Autodesk Fusion 360 part; units mm, degrees
(part 2 of 3)
  arc A296 (115.4627, 116.2428) -> (115.5827, 116.3629) centre (115.4627, 116.3629) ccw
  arc A297 (96.7858, 84.677) -> (96.862, 84.7532) centre (96.7858, 84.7532) ccw
  arc A298 (57.1697, 56.4515) -> (57.2897, 56.5715) centre (57.1697, 56.5715) ccw
  arc A299 (113.2577, 58.5983) -> (113.3777, 58.7183) centre (113.2577, 58.7183) ccw
  line L491 (67.31, 68.0838) -> (67.31, 67.2202)
  line L492 (57.2897, 59.4163) -> (57.2897, 60.7765)
  arc A300 (50.1015, 56.3683) -> (50.2215, 56.2483) centre (50.2215, 56.3683) ccw
  arc A301 (115.5827, 117.9262) -> (115.4627, 118.0462) centre (115.4627, 117.9262) ccw
  line L493 (115.5391, 123.5075) -> (113.9758, 123.5075)
  line L494 (113.9758, 119.0625) -> (115.5391, 119.0625)
  arc A302 (105.1869, 119.9007) -> (105.0668, 119.7807) centre (105.1869, 119.7807) ccw
  line L495 (50.1015, 57.9317) -> (50.1015, 56.3683)
  arc A303 (106.667, 119.7807) -> (106.547, 119.9007) centre (106.547, 119.7807) ccw
  line L496 (55.4863, 57.9317) -> (55.4863, 56.5715)
  line L497 (96.862, 84.7532) -> (96.862, 85.6168)
  arc A304 (105.0668, 118.2173) -> (105.1869, 118.0973) centre (105.1869, 118.2173) ccw
  arc A305 (115.5391, 119.0625) -> (115.6592, 119.1825) centre (115.5391, 119.1825) ccw
  arc A306 (68.326, 66.3838) -> (68.2498, 66.46) centre (68.2498, 66.3838) ccw
  arc A307 (113.9758, 120.6627) -> (113.8558, 120.5427) centre (113.9758, 120.5427) ccw
  line L498 (113.8558, 123.3875) -> (113.8558, 122.0273)
  line L499 (111.7775, 60.2817) -> (111.7775, 58.7183)
  line L500 (113.2577, 60.4017) -> (111.8975, 60.4017)
  line L501 (114.6223, 60.2817) -> (114.6223, 58.7183)
  arc A308 (95.846, 84.7532) -> (95.9222, 84.677) centre (95.9222, 84.7532) ccw
  line L502 (57.1697, 60.8965) -> (55.6063, 60.8965)
  line L503 (115.5827, 116.3629) -> (115.5827, 117.9262)
  line L504 (111.8975, 58.5983) -> (113.2577, 58.5983)
  line L505 (113.9825, 117.9262) -> (113.9825, 116.3629)
  line L506 (96.7858, 85.693) -> (95.9222, 85.693)
  line L507 (108.1532, 114.5165) -> (109.0168, 114.5165)
  arc A309 (57.2897, 57.9317) -> (57.1697, 58.0517) centre (57.1697, 57.9317) ccw
  line L508 (109.0168, 115.5325) -> (108.1532, 115.5325)
  arc A310 (111.8975, 60.4017) -> (111.7775, 60.2817) centre (111.8975, 60.2817) ccw
  arc A311 (95.9222, 85.693) -> (95.846, 85.6168) centre (95.9222, 85.6168) ccw
  line L509 (95.0858, 85.693) -> (94.2222, 85.693)
  arc A312 (113.9825, 116.3629) -> (114.1025, 116.2428) centre (114.1025, 116.3629) ccw
  line L510 (51.5817, 58.0517) -> (50.2215, 58.0517)
  arc A313 (115.5391, 121.9073) -> (115.6592, 122.0273) centre (115.5391, 122.0273) ccw
  line L511 (109.093, 114.5927) -> (109.093, 115.4563)
  arc A314 (108.1532, 115.5325) -> (108.077, 115.4563) centre (108.1532, 115.4563) ccw
  arc A315 (57.1697, 59.2963) -> (57.2897, 59.4163) centre (57.1697, 59.4163) ccw
  arc A316 (108.077, 114.5927) -> (108.1532, 114.5165) centre (108.1532, 114.5927) ccw
  arc A317 (109.0168, 114.5165) -> (109.093, 114.5927) centre (109.0168, 114.5927) ccw
  line L512 (95.846, 85.6168) -> (95.846, 84.7532)
  line L513 (118.4275, 116.3629) -> (118.4275, 117.9262)
  line L514 (57.2897, 56.5715) -> (57.2897, 57.9317)
  arc A318 (109.093, 115.4563) -> (109.0168, 115.5325) centre (109.0168, 115.4563) ccw
  arc A319 (96.862, 85.6168) -> (96.7858, 85.693) centre (96.7858, 85.6168) ccw
  arc A320 (95.0858, 84.677) -> (95.162, 84.7532) centre (95.0858, 84.7532) ccw
  arc A321 (55.6063, 60.8965) -> (55.4863, 60.7765) centre (55.6063, 60.7765) ccw
  arc A322 (57.2897, 60.7765) -> (57.1697, 60.8965) centre (57.1697, 60.7765) ccw
  arc A323 (116.9473, 118.0462) -> (116.8273, 117.9262) centre (116.9473, 117.9262) ccw
  line L515 (108.1532, 116.2165) -> (109.0168, 116.2165)
  arc A324 (68.2498, 67.144) -> (68.326, 67.2202) centre (68.2498, 67.2202) ccw
  arc A325 (94.146, 84.7532) -> (94.2222, 84.677) centre (94.2222, 84.7532) ccw
  line L516 (68.2498, 68.16) -> (67.3862, 68.16)
  arc A326 (67.31, 65.5202) -> (67.3862, 65.444) centre (67.3862, 65.5202) ccw
  arc A327 (55.6063, 58.0517) -> (55.4863, 57.9317) centre (55.6063, 57.9317) ccw
  arc A328 (111.6705, 112.3188) -> (111.5943, 112.395) centre (111.5943, 112.3188) ccw
  arc A329 (109.0168, 116.2165) -> (109.093, 116.2927) centre (109.0168, 116.2927) ccw
  line L517 (108.9545, 112.3188) -> (108.9545, 111.4552)
  arc A330 (55.4863, 59.4163) -> (55.6063, 59.2963) centre (55.6063, 59.4163) ccw
  line L518 (107.149, 112.3188) -> (107.149, 111.4552)
  line L519 (116.0662, 111.379) -> (116.9298, 111.379)
  line L520 (68.2498, 66.46) -> (67.3862, 66.46)
  arc A331 (117.006, 112.3188) -> (116.9298, 112.395) centre (116.9298, 112.3188) ccw
  line L521 (55.6063, 56.4515) -> (57.1697, 56.4515)
  line L522 (57.1697, 58.0517) -> (55.6063, 58.0517)
  arc A332 (108.1532, 117.2325) -> (108.077, 117.1563) centre (108.1532, 117.1563) ccw
  line L523 (118.706, 111.4552) -> (118.706, 112.3188)
  arc A333 (106.465, 112.3188) -> (106.3888, 112.395) centre (106.3888, 112.3188) ccw
  arc A334 (68.326, 68.0838) -> (68.2498, 68.16) centre (68.2498, 68.0838) ccw
  line L524 (50.2215, 56.2483) -> (51.5817, 56.2483)
  line L525 (95.9222, 84.677) -> (96.7858, 84.677)
  line L526 (55.4863, 60.7765) -> (55.4863, 59.4163)
  arc A335 (109.093, 117.1563) -> (109.0168, 117.2325) centre (109.0168, 117.1563) ccw
  arc A336 (51.7017, 57.9317) -> (51.5817, 58.0517) centre (51.5817, 57.9317) ccw
  line L527 (114.2361, 111.379) -> (115.0997, 111.379)
  line L528 (115.1759, 111.4552) -> (115.1759, 112.3188)
  arc A337 (67.3862, 68.16) -> (67.31, 68.0838) centre (67.3862, 68.0838) ccw
  arc A338 (51.5817, 56.2483) -> (51.7017, 56.3683) centre (51.5817, 56.3683) ccw
  line L529 (114.1599, 112.3188) -> (114.1599, 111.4552)
  arc A339 (67.31, 67.2202) -> (67.3862, 67.144) centre (67.3862, 67.2202) ccw
  arc A340 (115.0997, 111.379) -> (115.1759, 111.4552) centre (115.0997, 111.4552) ccw
  line L530 (108.077, 117.1563) -> (108.077, 116.2927)
  line L531 (67.31, 66.3838) -> (67.31, 65.5202)
  line L532 (94.146, 85.6168) -> (94.146, 84.7532)
  arc A341 (108.165, 112.3188) -> (108.0888, 112.395) centre (108.0888, 112.3188) ccw
  line L533 (109.9705, 111.4552) -> (109.9705, 112.3188)
  arc A342 (55.4863, 56.5715) -> (55.6063, 56.4515) centre (55.6063, 56.5715) ccw
  line L534 (68.326, 67.2202) -> (68.326, 68.0838)
  arc A343 (67.3862, 66.46) -> (67.31, 66.3838) centre (67.3862, 66.3838) ccw
  arc A344 (116.0662, 112.395) -> (115.99, 112.3188) centre (116.0662, 112.3188) ccw
  arc A345 (115.1759, 112.3188) -> (115.0997, 112.395) centre (115.0997, 112.3188) ccw
  arc A346 (114.1599, 111.4552) -> (114.2361, 111.379) centre (114.2361, 111.4552) ccw
  line L535 (110.7307, 111.379) -> (111.5943, 111.379)
  line L536 (55.6063, 59.2963) -> (57.1697, 59.2963)
  line L537 (107.2252, 111.379) -> (108.0888, 111.379)
  line L538 (117.7662, 111.379) -> (118.6298, 111.379)
  line L539 (67.3862, 65.444) -> (68.2498, 65.444)
  arc A347 (109.0307, 112.395) -> (108.9545, 112.3188) centre (109.0307, 112.3188) ccw
  line L540 (108.165, 111.4552) -> (108.165, 112.3188)
  arc A348 (94.2222, 85.693) -> (94.146, 85.6168) centre (94.2222, 85.6168) ccw
  line L541 (115.0997, 112.395) -> (114.2361, 112.395)
  arc A349 (68.2498, 65.444) -> (68.326, 65.5202) centre (68.2498, 65.5202) ccw
  line L542 (108.0888, 112.395) -> (107.2252, 112.395)
  line L543 (118.6298, 112.395) -> (117.7662, 112.395)
  arc A350 (114.2361, 112.395) -> (114.1599, 112.3188) centre (114.2361, 112.3188) ccw
  arc A351 (50.2215, 58.0517) -> (50.1015, 57.9317) centre (50.2215, 57.9317) ccw
  line L544 (115.99, 112.3188) -> (115.99, 111.4552)
  line L545 (117.006, 111.4552) -> (117.006, 112.3188)
  line L546 (116.9298, 112.395) -> (116.0662, 112.395)
  line L547 (109.0307, 111.379) -> (109.8943, 111.379)
  line L548 (95.162, 84.7532) -> (95.162, 85.6168)
  line L549 (105.5252, 111.379) -> (106.3888, 111.379)
  line L550 (68.326, 65.5202) -> (68.326, 66.3838)
  arc A352 (93.2688, 79.001) -> (93.345, 79.0772) centre (93.2688, 79.0772) ccw
  line L551 (105.449, 112.3188) -> (105.449, 111.4552)
  arc A353 (93.2688, 80.701) -> (93.345, 80.7772) centre (93.2688, 80.7772) ccw
  arc A354 (117.69, 111.4552) -> (117.7662, 111.379) centre (117.7662, 111.4552) ccw
  arc A355 (115.99, 111.4552) -> (116.0662, 111.379) centre (116.0662, 111.4552) ccw
  arc A356 (59.182, 50.4562) -> (59.2582, 50.38) centre (59.2582, 50.4562) ccw
  line L552 (109.093, 116.2927) -> (109.093, 117.1563)
  line L553 (113.4759, 111.4552) -> (113.4759, 112.3188)
  arc A357 (116.9298, 111.379) -> (117.006, 111.4552) centre (116.9298, 111.4552) ccw
  arc A358 (45.9622, 85.725) -> (45.886, 85.6488) centre (45.9622, 85.6488) ccw
  arc A359 (112.5361, 112.395) -> (112.4599, 112.3188) centre (112.5361, 112.3188) ccw
  arc A360 (113.4759, 112.3188) -> (113.3997, 112.395) centre (113.3997, 112.3188) ccw
  line L554 (106.465, 111.4552) -> (106.465, 112.3188)
  arc A361 (111.5943, 111.379) -> (111.6705, 111.4552) centre (111.5943, 111.4552) ccw
  line L555 (92.4052, 79.001) -> (93.2688, 79.001)
  arc A362 (93.345, 79.9408) -> (93.2688, 80.017) centre (93.2688, 79.9408) ccw
  arc A363 (60.1218, 50.38) -> (60.198, 50.4562) centre (60.1218, 50.4562) ccw
  arc A364 (105.449, 111.4552) -> (105.5252, 111.379) centre (105.5252, 111.4552) ccw
  line L556 (60.198, 48.7562) -> (60.198, 49.6198)
  arc A365 (118.706, 112.3188) -> (118.6298, 112.395) centre (118.6298, 112.3188) ccw
  line L557 (112.5361, 111.379) -> (113.3997, 111.379)
  line L558 (110.6545, 112.3188) -> (110.6545, 111.4552)
  arc A366 (109.9705, 112.3188) -> (109.8943, 112.395) centre (109.8943, 112.3188) ccw
  arc A367 (105.5252, 112.395) -> (105.449, 112.3188) centre (105.5252, 112.3188) ccw
  line L559 (47.586, 85.6488) -> (47.586, 84.7852)
  arc A368 (107.149, 111.4552) -> (107.2252, 111.379) centre (107.2252, 111.4552) ccw
  line L560 (92.329, 79.9408) -> (92.329, 79.0772)
  arc A369 (110.7307, 112.395) -> (110.6545, 112.3188) centre (110.7307, 112.3188) ccw
  arc A370 (48.5258, 84.709) -> (48.602, 84.7852) centre (48.5258, 84.7852) ccw
  line L561 (117.69, 112.3188) -> (117.69, 111.4552)
  arc A371 (108.077, 116.2927) -> (108.1532, 116.2165) centre (108.1532, 116.2927) ccw
  arc A372 (92.4052, 84.081) -> (92.329, 84.0048) centre (92.4052, 84.0048) ccw
  arc A373 (47.6622, 85.725) -> (47.586, 85.6488) centre (47.6622, 85.6488) ccw
  line L562 (92.329, 81.6408) -> (92.329, 80.7772)
  line L563 (60.1218, 51.396) -> (59.2582, 51.396)
  line L564 (93.345, 83.1412) -> (93.345, 84.0048)
  line L565 (59.2582, 50.38) -> (60.1218, 50.38)
  arc A374 (118.6298, 111.379) -> (118.706, 111.4552) centre (118.6298, 111.4552) ccw
  line L566 (111.5943, 112.395) -> (110.7307, 112.395)
  line L567 (109.8943, 112.395) -> (109.0307, 112.395)
  line L568 (92.329, 85.7048) -> (92.329, 84.8412)
  line L569 (93.345, 80.7772) -> (93.345, 81.6408)
  arc A375 (60.198, 51.3198) -> (60.1218, 51.396) centre (60.1218, 51.3198) ccw
  arc A376 (108.9545, 111.4552) -> (109.0307, 111.379) centre (109.0307, 111.4552) ccw
  arc A377 (110.6545, 111.4552) -> (110.7307, 111.379) centre (110.7307, 111.4552) ccw
  line L570 (47.6622, 84.709) -> (48.5258, 84.709)
  line L571 (109.0168, 117.2325) -> (108.1532, 117.2325)
  arc A378 (92.329, 84.8412) -> (92.4052, 84.765) centre (92.4052, 84.8412) ccw
  arc A379 (59.2582, 51.396) -> (59.182, 51.3198) centre (59.2582, 51.3198) ccw
  line L572 (111.6705, 111.4552) -> (111.6705, 112.3188)
  arc A380 (107.2252, 112.395) -> (107.149, 112.3188) centre (107.2252, 112.3188) ccw
  arc A381 (108.0888, 111.379) -> (108.165, 111.4552) centre (108.0888, 111.4552) ccw
  arc A382 (117.7662, 112.395) -> (117.69, 112.3188) centre (117.7662, 112.3188) ccw
  arc A383 (92.329, 80.7772) -> (92.4052, 80.701) centre (92.4052, 80.7772) ccw
  line L573 (46.902, 84.7852) -> (46.902, 85.6488)
  line L574 (59.182, 51.3198) -> (59.182, 50.4562)
  arc A384 (106.3888, 111.379) -> (106.465, 111.4552) centre (106.3888, 111.4552) ccw
  line L575 (60.198, 50.4562) -> (60.198, 51.3198)
  arc A385 (92.4052, 81.717) -> (92.329, 81.6408) centre (92.4052, 81.6408) ccw
  line L576 (106.3888, 112.395) -> (105.5252, 112.395)
  line L577 (93.2688, 81.717) -> (92.4052, 81.717)
  arc A386 (109.8943, 111.379) -> (109.9705, 111.4552) centre (109.8943, 111.4552) ccw
  line L578 (58.711, 77.262) -> (58.711, 76.662)
  line L579 (53.811, 77.262) -> (52.211, 77.262)
  line L580 (52.211, 77.262) -> (52.211, 76.662)
  arc A387 (105.456, 63.44) -> (104.856, 63.44) centre (105.156, 63.44) ccw
  line L581 (105.456, 57.24) -> (104.856, 57.24)
  line L582 (107.996, 57.24) -> (107.396, 57.24)
  line L583 (104.856, 57.24) -> (104.856, 55.64)
  line L584 (107.996, 55.64) -> (107.996, 57.24)
  line L585 (107.396, 57.24) -> (107.396, 55.64)
  line L586 (107.996, 63.74) -> (107.396, 63.74)
  line L587 (53.811, 76.662) -> (53.811, 77.262)
  line L588 (53.511, 74.722) -> (52.511, 74.722)
  line L589 (97.5478, 65.659) -> (96.6842, 65.659)
  line L590 (96.608, 65.5828) -> (96.608, 64.7192)
  line L591 (107.396, 55.64) -> (107.996, 55.64)
  arc A388 (96.608, 64.7192) -> (96.6842, 64.643) centre (96.6842, 64.7192) ccw
  line L592 (60.311, 77.262) -> (58.711, 77.262)
  line L593 (107.996, 62.14) -> (107.996, 63.74)
  line L594 (60.311, 74.122) -> (60.311, 74.722)
  line L595 (104.856, 62.44) -> (104.856, 63.44)
  line L596 (105.456, 62.44) -> (105.456, 63.44)
  line L597 (104.856, 55.64) -> (105.456, 55.64)
  line L598 (58.711, 74.122) -> (60.311, 74.122)
  line L599 (60.311, 74.722) -> (58.711, 74.722)
  line L600 (52.211, 76.662) -> (53.811, 76.662)
  arc A389 (52.511, 74.722) -> (52.511, 74.122) centre (52.511, 74.422) ccw
  line L601 (107.396, 62.14) -> (107.996, 62.14)
  line L602 (107.396, 63.74) -> (107.396, 62.14)
  line L603 (105.456, 55.64) -> (105.456, 57.24)
  line L604 (58.711, 74.722) -> (58.711, 74.122)
  line L605 (106.0078, 65.532) -> (105.1442, 65.532)
  line L606 (97.624, 64.7192) -> (97.624, 65.5828)
  arc A390 (94.322, 65.5828) -> (94.2458, 65.659) centre (94.2458, 65.5828) ccw
  arc A391 (97.5478, 64.643) -> (97.624, 64.7192) centre (97.5478, 64.7192) ccw
  line L607 (91.6822, 64.643) -> (92.5458, 64.643)
  arc A392 (94.9842, 65.659) -> (94.908, 65.5828) centre (94.9842, 65.5828) ccw
  line L608 (105.1442, 64.516) -> (106.0078, 64.516)
  arc A393 (106.768, 64.5922) -> (106.8442, 64.516) centre (106.8442, 64.5922) ccw
  line L609 (104.355, 64.5922) -> (104.355, 65.4558)
  line L610 (93.306, 65.5828) -> (93.306, 64.7192)
  line L611 (103.4152, 64.516) -> (104.2788, 64.516)
  arc A394 (106.084, 65.4558) -> (106.0078, 65.532) centre (106.0078, 65.4558) ccw
  line L612 (92.5458, 65.659) -> (91.6822, 65.659)
  arc A395 (91.606, 64.7192) -> (91.6822, 64.643) centre (91.6822, 64.7192) ccw
  arc A396 (92.622, 65.5828) -> (92.5458, 65.659) centre (92.5458, 65.5828) ccw
  arc A397 (95.8478, 64.643) -> (95.924, 64.7192) centre (95.8478, 64.7192) ccw
  line L613 (106.8442, 64.516) -> (107.7078, 64.516)
  line L614 (107.784, 64.5922) -> (107.784, 65.4558)
  arc A398 (107.7078, 64.516) -> (107.784, 64.5922) centre (107.7078, 64.5922) ccw
  arc A399 (97.624, 65.5828) -> (97.5478, 65.659) centre (97.5478, 65.5828) ccw
  arc A400 (93.306, 64.7192) -> (93.3822, 64.643) centre (93.3822, 64.7192) ccw
  arc A401 (94.908, 64.7192) -> (94.9842, 64.643) centre (94.9842, 64.7192) ccw
  line L615 (94.908, 65.5828) -> (94.908, 64.7192)
  arc A402 (106.8442, 65.532) -> (106.768, 65.4558) centre (106.8442, 65.4558) ccw
  arc A403 (95.924, 65.5828) -> (95.8478, 65.659) centre (95.8478, 65.5828) ccw
  line L616 (103.339, 65.4558) -> (103.339, 64.5922)
  arc A404 (106.0078, 64.516) -> (106.084, 64.5922) centre (106.0078, 64.5922) ccw
  line L617 (94.2458, 65.659) -> (93.3822, 65.659)
  line L618 (95.8478, 65.659) -> (94.9842, 65.659)
  line L619 (93.3822, 64.643) -> (94.2458, 64.643)
  line L620 (104.2788, 65.532) -> (103.4152, 65.532)
  arc A405 (96.6842, 65.659) -> (96.608, 65.5828) centre (96.6842, 65.5828) ccw
  line L621 (101.639, 65.4558) -> (101.639, 64.5922)
  arc A406 (93.3822, 65.659) -> (93.306, 65.5828) centre (93.3822, 65.5828) ccw
  arc A407 (103.339, 64.5922) -> (103.4152, 64.516) centre (103.4152, 64.5922) ccw
  arc A408 (102.655, 65.4558) -> (102.5788, 65.532) centre (102.5788, 65.4558) ccw
  arc A409 (94.2458, 64.643) -> (94.322, 64.7192) centre (94.2458, 64.7192) ccw
  line L622 (94.322, 64.7192) -> (94.322, 65.5828)
  line L623 (92.622, 64.7192) -> (92.622, 65.5828)
  line L624 (102.5788, 65.532) -> (101.7152, 65.532)
  arc A410 (105.1442, 65.532) -> (105.068, 65.4558) centre (105.1442, 65.4558) ccw
  arc A411 (101.639, 64.5922) -> (101.7152, 64.516) centre (101.7152, 64.5922) ccw
  line L625 (94.9842, 64.643) -> (95.8478, 64.643)
  arc A412 (107.784, 65.4558) -> (107.7078, 65.532) centre (107.7078, 65.4558) ccw
  line L626 (101.7152, 64.516) -> (102.5788, 64.516)
  arc A413 (91.6822, 65.659) -> (91.606, 65.5828) centre (91.6822, 65.5828) ccw
  arc A414 (104.2788, 64.516) -> (104.355, 64.5922) centre (104.2788, 64.5922) ccw
  line L627 (95.141, 48.71) -> (94.741, 49.11)
  line L628 (107.7078, 65.532) -> (106.8442, 65.532)
  arc A415 (104.355, 65.4558) -> (104.2788, 65.532) centre (104.2788, 65.4558) ccw
  line L629 (91.606, 65.5828) -> (91.606, 64.7192)
  line L630 (102.655, 64.5922) -> (102.655, 65.4558)
  arc A416 (105.068, 64.5922) -> (105.1442, 64.516) centre (105.1442, 64.5922) ccw
  arc A417 (103.4152, 65.532) -> (103.339, 65.4558) centre (103.4152, 65.4558) ccw
  line L631 (95.924, 64.7192) -> (95.924, 65.5828)
  arc A418 (101.7152, 65.532) -> (101.639, 65.4558) centre (101.7152, 65.4558) ccw
  line L632 (105.068, 65.4558) -> (105.068, 64.5922)
  line L633 (106.768, 65.4558) -> (106.768, 64.5922)
  arc A419 (92.5458, 64.643) -> (92.622, 64.7192) centre (92.5458, 64.7192) ccw
  line L634 (106.084, 64.5922) -> (106.084, 65.4558)
  line L635 (96.6842, 64.643) -> (97.5478, 64.643)
  arc A420 (51.8042, 50.419) -> (51.728, 50.3428) centre (51.8042, 50.3428) ccw
  line L636 (55.303, 51.1585) -> (55.5155, 50.946)
  line L637 (55.9905, 51.796) -> (55.5155, 51.796)
  line L638 (55.303, 51.5835) -> (55.303, 51.1585)
  line L639 (55.5155, 50.946) -> (55.9905, 50.946)
  line L640 (93.941, 49.11) -> (93.541, 48.71)
  line L641 (93.941, 47.41) -> (94.741, 47.41)
  line L642 (55.9905, 50.946) -> (56.203, 51.1585)
  line L643 (56.203, 51.1585) -> (56.203, 51.5835)
  line L644 (109.151, 47.41) -> (109.151, 49.11)
  line L645 (116.389, 67.157) -> (116.389, 70.257)
  line L646 (97.391, 49.11) -> (97.391, 47.41)
  line L647 (93.541, 47.81) -> (93.941, 47.41)
  line L648 (52.6678, 50.419) -> (51.8042, 50.419)
  line L649 (51.728, 50.3428) -> (51.728, 49.4792)
  line L650 (93.541, 48.71) -> (93.541, 47.81)
  arc A421 (53.428, 49.4792) -> (53.5042, 49.403) centre (53.5042, 49.4792) ccw
  arc A422 (51.728, 49.4792) -> (51.8042, 49.403) centre (51.8042, 49.4792) ccw
  line L651 (54.444, 49.4792) -> (54.444, 50.3428)
  line L652 (107.551, 47.41) -> (109.151, 47.41)
  line L653 (104.101, 47.41) -> (104.901, 47.41)
  line L654 (52.744, 49.4792) -> (52.744, 50.3428)
  line L655 (51.8042, 49.403) -> (52.6678, 49.403)
  arc A423 (52.6678, 49.403) -> (52.744, 49.4792) centre (52.6678, 49.4792) ccw
  arc A424 (54.444, 50.3428) -> (54.3678, 50.419) centre (54.3678, 50.3428) ccw
  line L656 (103.701, 48.71) -> (103.701, 47.81)
  line L657 (95.141, 47.81) -> (95.141, 48.71)
  arc A425 (53.5042, 50.419) -> (53.428, 50.3428) centre (53.5042, 50.3428) ccw
  line L658 (55.303, 49.296) -> (56.203, 49.296)
  line L659 (55.303, 50.146) -> (55.303, 49.296)
  line L660 (55.5155, 51.796) -> (55.303, 51.5835)
  line L661 (54.3678, 50.419) -> (53.5042, 50.419)
  line L662 (113.989, 70.257) -> (113.989, 67.157)
  arc A426 (54.3678, 49.403) -> (54.444, 49.4792) centre (54.3678, 49.4792) ccw
  line L663 (104.901, 47.41) -> (105.301, 47.81)
  arc A427 (102.5788, 64.516) -> (102.655, 64.5922) centre (102.5788, 64.5922) ccw
  line L664 (94.741, 49.11) -> (93.941, 49.11)
  line L665 (117.014, 69.642) -> (117.014, 69.042)
  line L666 (53.428, 50.3428) -> (53.428, 49.4792)
  line L667 (118.764, 70.312) -> (118.764, 70.912)
  line L668 (118.764, 69.642) -> (117.014, 69.642)
  line L669 (117.014, 69.042) -> (118.764, 69.042)
  line L670 (113.989, 67.157) -> (116.389, 67.157)
  line L671 (118.764, 70.912) -> (117.014, 70.912)
  line L672 (53.5042, 49.403) -> (54.3678, 49.403)
  line L673 (103.701, 47.81) -> (104.101, 47.41)
  line L674 (98.991, 49.11) -> (97.391, 49.11)
  line L675 (56.203, 51.5835) -> (55.9905, 51.796)
  line L676 (56.203, 50.146) -> (55.303, 50.146)
  line L677 (98.991, 47.41) -> (98.991, 49.11)
  line L678 (97.391, 47.41) -> (98.991, 47.41)
  line L679 (117.014, 70.912) -> (117.014, 70.312)
  line L680 (105.301, 48.71) -> (104.901, 49.11)
  line L681 (107.551, 49.11) -> (107.551, 47.41)
  line L682 (118.764, 69.042) -> (118.764, 69.642)
  line L683 (116.389, 70.257) -> (113.989, 70.257)
  line L684 (109.151, 49.11) -> (107.551, 49.11)
  line L685 (104.901, 49.11) -> (104.101, 49.11)
  line L686 (56.203, 49.296) -> (56.203, 50.146)
  line L687 (117.014, 70.312) -> (118.764, 70.312)
  line L688 (104.101, 49.11) -> (103.701, 48.71)
  arc A428 (52.744, 50.3428) -> (52.6678, 50.419) centre (52.6678, 50.3428) ccw
  line L689 (105.301, 47.81) -> (105.301, 48.71)
  line L690 (94.741, 47.41) -> (95.141, 47.81)
  arc A429 (93.0402, 70.954) -> (92.964, 70.8778) centre (93.0402, 70.8778) ccw
  line L691 (118.764, 67.102) -> (117.014, 67.102)
  line L692 (111.614, 68.372) -> (111.614, 67.772)
  line L693 (111.614, 70.912) -> (111.614, 70.312)
  line L694 (113.064, 66.502) -> (111.914, 66.502)
  line L695 (111.614, 70.312) -> (113.364, 70.312)
  line L696 (40.008, 63.7182) -> (40.008, 64.5818)
  line L697 (39.0682, 65.342) -> (39.9318, 65.342)
  arc A430 (39.9318, 65.342) -> (40.008, 65.4182) centre (39.9318, 65.4182) ccw
  line L698 (40.992, 66.2818) -> (40.992, 65.4182)
  line L699 (97.236, 63.74) -> (97.236, 62.14)
  line L700 (95.296, 57.24) -> (94.696, 57.24)
  line L701 (113.364, 68.372) -> (111.614, 68.372)
  line L702 (93.98, 70.0142) -> (93.98, 70.8778)
  line L703 (97.836, 62.14) -> (97.836, 63.74)
  line L704 (117.014, 67.772) -> (118.764, 67.772)
  arc A431 (42.008, 66.2818) -> (41.9318, 66.358) centre (41.9318, 66.2818) ccw
  line L705 (40.008, 65.4182) -> (40.008, 66.2818)
  arc A432 (40.992, 63.7182) -> (41.0682, 63.642) centre (41.0682, 63.7182) ccw
  line L706 (113.364, 70.912) -> (111.614, 70.912)
  line L707 (111.614, 69.642) -> (111.614, 69.042)
  line L708 (113.364, 69.042) -> (113.364, 69.642)
  arc A433 (53.511, 74.122) -> (53.511, 74.722) centre (53.511, 74.422) ccw
  line L709 (38.992, 66.2818) -> (38.992, 65.4182)
  line L710 (118.764, 66.502) -> (118.764, 67.102)
  line L711 (39.9318, 66.358) -> (39.0682, 66.358)
  line L712 (39.0682, 63.642) -> (39.9318, 63.642)
  line L713 (111.614, 69.042) -> (113.364, 69.042)
  line L714 (118.764, 67.772) -> (118.764, 68.372)
  line L715 (53.511, 74.122) -> (52.511, 74.122)
  line L716 (117.014, 66.502) -> (118.764, 66.502)
  arc A434 (39.0682, 66.358) -> (38.992, 66.2818) centre (39.0682, 66.2818) ccw
  line L717 (118.764, 68.372) -> (117.014, 68.372)
  line L718 (113.064, 67.102) -> (111.914, 67.102)
  line L719 (111.614, 67.772) -> (113.364, 67.772)
  line L720 (41.9318, 64.658) -> (41.0682, 64.658)
  line L721 (40.992, 64.5818) -> (40.992, 63.7182)
  line L722 (113.364, 69.642) -> (111.614, 69.642)
  line L723 (113.364, 70.312) -> (113.364, 70.912)
  line L724 (39.9318, 64.658) -> (39.0682, 64.658)
  line L725 (58.711, 76.662) -> (60.311, 76.662)
  line L726 (38.992, 64.5818) -> (38.992, 63.7182)
  arc A435 (40.008, 64.5818) -> (39.9318, 64.658) centre (39.9318, 64.5818) ccw
  line L727 (42.008, 63.7182) -> (42.008, 64.5818)
  line L728 (117.014, 68.372) -> (117.014, 67.772)
  arc A436 (40.008, 66.2818) -> (39.9318, 66.358) centre (39.9318, 66.2818) ccw
  line L729 (41.0682, 63.642) -> (41.9318, 63.642)
  line L730 (42.008, 65.4182) -> (42.008, 66.2818)
  line L731 (41.9318, 66.358) -> (41.0682, 66.358)
  arc A437 (111.914, 67.102) -> (111.914, 66.502) centre (111.914, 66.802) ccw
  arc A438 (41.0682, 66.358) -> (40.992, 66.2818) centre (41.0682, 66.2818) ccw
  arc A439 (113.064, 66.502) -> (113.064, 67.102) centre (113.064, 66.802) ccw
  line L732 (113.364, 67.772) -> (113.364, 68.372)
  arc A440 (38.992, 63.7182) -> (39.0682, 63.642) centre (39.0682, 63.7182) ccw
  arc A441 (38.992, 65.4182) -> (39.0682, 65.342) centre (39.0682, 65.4182) ccw
  line L733 (93.9038, 69.254) -> (93.0402, 69.254)
  arc A442 (93.98, 69.1778) -> (93.9038, 69.254) centre (93.9038, 69.1778) ccw
  arc A443 (95.296, 63.44) -> (94.696, 63.44) centre (94.996, 63.44) ccw
  arc A444 (39.0682, 64.658) -> (38.992, 64.5818) centre (39.0682, 64.5818) ccw
  arc A445 (41.0682, 64.658) -> (40.992, 64.5818) centre (41.0682, 64.5818) ccw
  line L734 (94.696, 55.64) -> (95.296, 55.64)
  arc A446 (39.9318, 63.642) -> (40.008, 63.7182) centre (39.9318, 63.7182) ccw
  arc A447 (41.9318, 65.342) -> (42.008, 65.4182) centre (41.9318, 65.4182) ccw
  line L735 (117.014, 67.102) -> (117.014, 66.502)
  arc A448 (61.722, 77.2532) -> (61.7982, 77.177) centre (61.7982, 77.2532) ccw
  line L736 (97.9873, 90.955) -> (97.8373, 91.105)
  line L737 (41.0682, 65.342) -> (41.9318, 65.342)
  line L738 (94.696, 62.44) -> (94.696, 63.44)
  line L739 (108.2873, 93.045) -> (108.2873, 93.645)
  line L740 (106.2373, 90.505) -> (108.2873, 90.505)
  line L741 (58.711, 80.98) -> (60.311, 80.98)
  arc A449 (61.722, 75.5532) -> (61.7982, 75.477) centre (61.7982, 75.5532) ccw
  line L742 (97.8373, 91.105) -> (96.0873, 91.105)
  line L743 (53.811, 84.12) -> (52.211, 84.12)
  line L744 (53.511, 80.98) -> (52.511, 80.98)
  line L745 (97.236, 57.24) -> (97.236, 55.64)
  arc A450 (92.964, 68.3142) -> (93.0402, 68.238) centre (93.0402, 68.3142) ccw
  line L746 (93.0402, 69.938) -> (93.9038, 69.938)
  arc A451 (104.856, 62.44) -> (105.456, 62.44) centre (105.156, 62.44) ccw
  line L747 (108.2873, 93.645) -> (106.2373, 93.645)
  line L748 (61.722, 76.4168) -> (61.722, 75.5532)
  arc A452 (61.7982, 76.493) -> (61.722, 76.4168) centre (61.7982, 76.4168) ccw
  arc A453 (52.511, 81.58) -> (52.511, 80.98) centre (52.511, 81.28) ccw
  line L749 (62.738, 77.2532) -> (62.738, 78.1168)
  arc A454 (62.6618, 75.477) -> (62.738, 75.5532) centre (62.6618, 75.5532) ccw
  line L750 (94.696, 57.24) -> (94.696, 55.64)
  line L751 (60.311, 81.58) -> (58.711, 81.58)
  arc A455 (62.738, 76.4168) -> (62.6618, 76.493) centre (62.6618, 76.4168) ccw
  line L752 (97.836, 57.24) -> (97.236, 57.24)
  line L753 (97.836, 55.64) -> (97.836, 57.24)
  line L754 (97.9873, 90.655) -> (97.9873, 90.955)
  line L755 (96.0873, 91.105) -> (95.9373, 90.955)
  line L756 (95.296, 55.64) -> (95.296, 57.24)
  line L757 (93.0402, 68.238) -> (93.9038, 68.238)
  line L758 (61.7982, 77.177) -> (62.6618, 77.177)
  arc A456 (93.9038, 69.938) -> (93.98, 70.0142) centre (93.9038, 70.0142) ccw
  arc A457 (53.511, 80.98) -> (53.511, 81.58) centre (53.511, 81.28) ccw
  line L759 (93.98, 68.3142) -> (93.98, 69.1778)
  line L760 (62.738, 75.5532) -> (62.738, 76.4168)
  line L761 (95.9373, 90.955) -> (95.9373, 90.655)
  arc A458 (93.9038, 68.238) -> (93.98, 68.3142) centre (93.9038, 68.3142) ccw
  arc A459 (93.98, 70.8778) -> (93.9038, 70.954) centre (93.9038, 70.8778) ccw
  line L762 (93.9038, 70.954) -> (93.0402, 70.954)
  line L763 (61.7982, 75.477) -> (62.6618, 75.477)
  arc A460 (41.9318, 63.642) -> (42.008, 63.7182) centre (41.9318, 63.7182) ccw
  arc A461 (40.992, 65.4182) -> (41.0682, 65.342) centre (41.0682, 65.4182) ccw
  line L764 (97.236, 55.64) -> (97.836, 55.64)
  line L765 (95.296, 62.44) -> (95.296, 63.44)
  line L766 (92.964, 70.8778) -> (92.964, 70.0142)
  arc A462 (42.008, 64.5818) -> (41.9318, 64.658) centre (41.9318, 64.5818) ccw
  arc A463 (94.696, 62.44) -> (95.296, 62.44) centre (94.996, 62.44) ccw
  line L767 (60.311, 80.98) -> (60.311, 81.58)
  line L768 (95.9373, 93.045) -> (97.9873, 93.045)
  line L769 (106.2373, 91.775) -> (108.2873, 91.775)
  line L770 (62.6618, 76.493) -> (61.7982, 76.493)
  line L771 (53.511, 81.58) -> (52.511, 81.58)
  arc A464 (92.964, 70.0142) -> (93.0402, 69.938) centre (93.0402, 70.0142) ccw
  line L772 (97.9873, 92.375) -> (95.9373, 92.375)
  line L773 (97.8373, 90.505) -> (97.9873, 90.655)
  line L774 (97.836, 63.74) -> (97.236, 63.74)
  line L775 (62.6618, 78.193) -> (61.7982, 78.193)
  arc A465 (62.6618, 77.177) -> (62.738, 77.2532) centre (62.6618, 77.2532) ccw
  line L776 (97.236, 62.14) -> (97.836, 62.14)
  line L777 (95.9373, 90.655) -> (96.0873, 90.505)
  line L778 (92.964, 69.1778) -> (92.964, 68.3142)
  line L779 (108.2873, 91.775) -> (108.2873, 92.375)
  arc A466 (93.0402, 69.254) -> (92.964, 69.1778) centre (93.0402, 69.1778) ccw
  line L780 (52.211, 84.12) -> (52.211, 83.52)
  line L781 (53.811, 83.52) -> (53.811, 84.12)
  arc A467 (66.4092, 74.295) -> (66.333, 74.2188) centre (66.4092, 74.2188) ccw
  line L782 (62.396, 74.3458) -> (62.396, 73.4822)
  line L783 (68.1092, 73.279) -> (68.9728, 73.279)
  line L784 (58.711, 81.58) -> (58.711, 80.98)
  line L785 (97.9873, 93.645) -> (95.9373, 93.645)
  arc A468 (49.4792, 77.05) -> (49.403, 76.9738) centre (49.4792, 76.9738) ccw
  arc A469 (50.3428, 76.034) -> (50.419, 76.1102) centre (50.3428, 76.1102) ccw
  line L786 (65.112, 73.4822) -> (65.112, 74.3458)
  line L787 (108.2873, 91.105) -> (106.2373, 91.105)
  arc A470 (62.4722, 74.422) -> (62.396, 74.3458) centre (62.4722, 74.3458) ccw
  line L788 (63.3358, 74.422) -> (62.4722, 74.422)
  line L789 (106.2373, 93.645) -> (106.2373, 93.045)
  line L790 (97.9873, 93.045) -> (97.9873, 93.645)
  line L791 (96.0873, 90.505) -> (97.8373, 90.505)
  line L792 (108.2873, 92.375) -> (106.2373, 92.375)
  line L793 (60.311, 76.662) -> (60.311, 77.262)
  arc A471 (62.738, 78.1168) -> (62.6618, 78.193) centre (62.6618, 78.1168) ccw
  line L794 (106.2373, 93.045) -> (108.2873, 93.045)
  line L795 (95.9373, 91.775) -> (97.9873, 91.775)
  line L796 (95.9373, 93.645) -> (95.9373, 93.045)
  line L797 (63.412, 73.4822) -> (63.412, 74.3458)
  line L798 (52.211, 83.52) -> (53.811, 83.52)
  line L799 (68.9728, 74.295) -> (68.1092, 74.295)
  arc A472 (50.3428, 74.334) -> (50.419, 74.4102) centre (50.3428, 74.4102) ccw
  line L800 (50.419, 74.4102) -> (50.419, 75.2738)
  arc A473 (62.396, 73.4822) -> (62.4722, 73.406) centre (62.4722, 73.4822) ccw
  line L801 (60.311, 83.52) -> (60.311, 84.12)
  line L802 (44.6278, 76.923) -> (43.7642, 76.923)
  arc A474 (68.033, 73.3552) -> (68.1092, 73.279) centre (68.1092, 73.3552) ccw
  line L803 (65.0358, 74.422) -> (64.1722, 74.422)
  arc A475 (50.419, 76.9738) -> (50.3428, 77.05) centre (50.3428, 76.9738) ccw
  arc A476 (43.688, 74.2832) -> (43.7642, 74.207) centre (43.7642, 74.2832) ccw
  arc A477 (50.419, 75.2738) -> (50.3428, 75.35) centre (50.3428, 75.2738) ccw
  arc A478 (64.1722, 74.422) -> (64.096, 74.3458) centre (64.1722, 74.3458) ccw
  line L804 (62.4722, 73.406) -> (63.3358, 73.406)
  line L805 (44.6278, 75.223) -> (43.7642, 75.223)
  line L806 (97.9873, 91.775) -> (97.9873, 92.375)
  line L807 (44.704, 74.2832) -> (44.704, 75.1468)
  line L808 (67.349, 73.3552) -> (67.349, 74.2188)
  arc A479 (65.0358, 73.406) -> (65.112, 73.4822) centre (65.0358, 73.4822) ccw
  arc A480 (43.7642, 76.923) -> (43.688, 76.8468) centre (43.7642, 76.8468) ccw
  line L809 (67.2728, 74.295) -> (66.4092, 74.295)
  line L810 (69.049, 73.3552) -> (69.049, 74.2188)
  arc A481 (49.4792, 75.35) -> (49.403, 75.2738) centre (49.4792, 75.2738) ccw
  arc A482 (61.7982, 78.193) -> (61.722, 78.1168) centre (61.7982, 78.1168) ccw
  line L811 (50.3428, 77.05) -> (49.4792, 77.05)
  line L812 (106.2373, 91.105) -> (106.2373, 90.505)
  arc A483 (43.688, 75.9832) -> (43.7642, 75.907) centre (43.7642, 75.9832) ccw
  arc A484 (44.704, 75.1468) -> (44.6278, 75.223) centre (44.6278, 75.1468) ccw
  line L813 (108.2873, 90.505) -> (108.2873, 91.105)
  arc A485 (43.7642, 75.223) -> (43.688, 75.1468) centre (43.7642, 75.1468) ccw
  line L814 (60.311, 84.12) -> (58.711, 84.12)
  arc A486 (44.6278, 74.207) -> (44.704, 74.2832) centre (44.6278, 74.2832) ccw
  arc A487 (67.349, 74.2188) -> (67.2728, 74.295) centre (67.2728, 74.2188) ccw
  line L815 (68.033, 74.2188) -> (68.033, 73.3552)
  arc A488 (68.9728, 73.279) -> (69.049, 73.3552) centre (68.9728, 73.3552) ccw
  line L816 (50.3428, 75.35) -> (49.4792, 75.35)
  line L817 (50.419, 76.1102) -> (50.419, 76.9738)
  line L818 (106.2373, 92.375) -> (106.2373, 91.775)
  line L819 (58.711, 83.52) -> (60.311, 83.52)
  line L820 (58.711, 84.12) -> (58.711, 83.52)
  line L821 (61.722, 78.1168) -> (61.722, 77.2532)
  line L822 (95.9373, 92.375) -> (95.9373, 91.775)
  line L823 (47.5352, 75.946) -> (48.3988, 75.946)
  arc A489 (48.475, 76.8858) -> (48.3988, 76.962) centre (48.3988, 76.8858) ccw
  line L824 (43.7642, 75.907) -> (44.6278, 75.907)
  arc A490 (63.412, 74.3458) -> (63.3358, 74.422) centre (63.3358, 74.3458) ccw
  arc A491 (63.3358, 73.406) -> (63.412, 73.4822) centre (63.3358, 73.4822) ccw
  line L825 (62.1538, 72.185) -> (61.2902, 72.185)
  arc A492 (45.8352, 76.962) -> (45.759, 76.8858) centre (45.8352, 76.8858) ccw
  arc A493 (47.5352, 76.962) -> (47.459, 76.8858) centre (47.5352, 76.8858) ccw
  line L826 (43.688, 76.8468) -> (43.688, 75.9832)
  arc A494 (46.6988, 75.946) -> (46.775, 76.0222) centre (46.6988, 76.0222) ccw
  arc A495 (62.1538, 71.169) -> (62.23, 71.2452) centre (62.1538, 71.2452) ccw
  arc A496 (78.8162, 59.69) -> (78.74, 59.6138) centre (78.8162, 59.6138) ccw
  arc A497 (70.397, 78.6892) -> (70.4732, 78.613) centre (70.4732, 78.6892) ccw
  arc A498 (66.333, 73.3552) -> (66.4092, 73.279) centre (66.4092, 73.3552) ccw
  line L827 (62.23, 71.2452) -> (62.23, 72.1088)
  line L828 (46.6988, 76.962) -> (45.8352, 76.962)
  arc A499 (69.049, 74.2188) -> (68.9728, 74.295) centre (68.9728, 74.2188) ccw
  arc A500 (64.096, 73.4822) -> (64.1722, 73.406) centre (64.1722, 73.4822) ccw
  arc A501 (61.2902, 70.485) -> (61.214, 70.4088) centre (61.2902, 70.4088) ccw
  line L829 (71.413, 78.6892) -> (71.413, 79.5528)
  line L830 (79.756, 58.7502) -> (79.756, 59.6138)
  line L831 (61.214, 70.4088) -> (61.214, 69.5452)
  arc A502 (65.112, 74.3458) -> (65.0358, 74.422) centre (65.0358, 74.3458) ccw
  arc A503 (72.1732, 79.629) -> (72.097, 79.5528) centre (72.1732, 79.5528) ccw
  line L832 (72.097, 79.5528) -> (72.097, 78.6892)
  arc A504 (61.2902, 72.185) -> (61.214, 72.1088) centre (61.2902, 72.1088) ccw
  line L833 (71.3368, 79.629) -> (70.4732, 79.629)
  arc A505 (44.704, 76.8468) -> (44.6278, 76.923) centre (44.6278, 76.8468) ccw
  line L834 (78.056, 58.7502) -> (78.056, 59.6138)
  line L835 (49.403, 76.9738) -> (49.403, 76.1102)
  line L836 (45.8352, 75.946) -> (46.6988, 75.946)
  arc A506 (78.74, 58.7502) -> (78.8162, 58.674) centre (78.8162, 58.7502) ccw
  arc A507 (68.1092, 74.295) -> (68.033, 74.2188) centre (68.1092, 74.2188) ccw
  arc A508 (67.2728, 73.279) -> (67.349, 73.3552) centre (67.2728, 73.3552) ccw
  line L837 (62.23, 69.5452) -> (62.23, 70.4088)
  arc A509 (62.1538, 69.469) -> (62.23, 69.5452) centre (62.1538, 69.5452) ccw
  line L838 (78.8162, 58.674) -> (79.6798, 58.674)
  arc A510 (61.214, 69.5452) -> (61.2902, 69.469) centre (61.2902, 69.5452) ccw
  arc A511 (45.759, 76.0222) -> (45.8352, 75.946) centre (45.8352, 76.0222) ccw
  line L839 (73.113, 78.6892) -> (73.113, 79.5528)
  arc A512 (73.0368, 78.613) -> (73.113, 78.6892) centre (73.0368, 78.6892) ccw
  arc A513 (78.056, 59.6138) -> (77.9798, 59.69) centre (77.9798, 59.6138) ccw
  line L840 (43.7642, 74.207) -> (44.6278, 74.207)
  arc A514 (49.403, 76.1102) -> (49.4792, 76.034) centre (49.4792, 76.1102) ccw
  arc A515 (61.214, 71.2452) -> (61.2902, 71.169) centre (61.2902, 71.2452) ccw
  line L841 (66.4092, 73.279) -> (67.2728, 73.279)
  line L842 (64.1722, 73.406) -> (65.0358, 73.406)
  arc A516 (48.3988, 75.946) -> (48.475, 76.0222) centre (48.3988, 76.0222) ccw
  line L843 (45.759, 76.8858) -> (45.759, 76.0222)
  line L844 (64.096, 74.3458) -> (64.096, 73.4822)
  line L845 (62.1538, 70.485) -> (61.2902, 70.485)
  line L846 (43.688, 75.1468) -> (43.688, 74.2832)
  line L847 (49.4792, 76.034) -> (50.3428, 76.034)
  line L848 (66.333, 74.2188) -> (66.333, 73.3552)
  line L849 (49.4792, 74.334) -> (50.3428, 74.334)
  arc A517 (49.403, 74.4102) -> (49.4792, 74.334) centre (49.4792, 74.4102) ccw
  line L850 (44.704, 75.9832) -> (44.704, 76.8468)
  arc A518 (44.6278, 75.907) -> (44.704, 75.9832) centre (44.6278, 75.9832) ccw
  line L851 (61.2902, 71.169) -> (62.1538, 71.169)
  line L852 (49.403, 75.2738) -> (49.403, 74.4102)
  line L853 (77.1162, 58.674) -> (77.9798, 58.674)
  arc A519 (46.775, 76.8858) -> (46.6988, 76.962) centre (46.6988, 76.8858) ccw
  arc A520 (77.1162, 59.69) -> (77.04, 59.6138) centre (77.1162, 59.6138) ccw
  arc A521 (47.459, 76.0222) -> (47.5352, 75.946) centre (47.5352, 76.0222) ccw
  line L854 (77.04, 59.6138) -> (77.04, 58.7502)
  line L855 (76.62, 74.8538) -> (76.62, 73.9902)
  arc A522 (58.028, 59.452) -> (58.133, 59.347) centre (58.133, 59.452) ccw
  line L856 (72.8862, 58.674) -> (73.7498, 58.674)
  line L857 (78.3962, 73.914) -> (79.2598, 73.914)
  line L858 (79.2598, 74.93) -> (78.3962, 74.93)
  arc A523 (59.828, 60.642) -> (59.723, 60.747) centre (59.723, 60.642) ccw
  arc A524 (70.016, 68.0838) -> (69.9398, 68.16) centre (69.9398, 68.0838) ccw
  arc A525 (78.32, 73.9902) -> (78.3962, 73.914) centre (78.3962, 73.9902) ccw
  arc A526 (79.336, 74.8538) -> (79.2598, 74.93) centre (79.2598, 74.8538) ccw
  arc A527 (77.636, 74.8538) -> (77.5598, 74.93) centre (77.5598, 74.8538) ccw
  arc A528 (69.9398, 67.144) -> (70.016, 67.2202) centre (69.9398, 67.2202) ccw
  arc A529 (62.23, 70.4088) -> (62.1538, 70.485) centre (62.1538, 70.4088) ccw
  arc A530 (71.413, 79.5528) -> (71.3368, 79.629) centre (71.3368, 79.5528) ccw
  line L859 (61.214, 72.1088) -> (61.214, 71.2452)
  arc A531 (69.9398, 65.444) -> (70.016, 65.5202) centre (69.9398, 65.5202) ccw
  line L860 (70.016, 67.2202) -> (70.016, 68.0838)
  line L861 (77.636, 73.9902) -> (77.636, 74.8538)
  arc A532 (74.5862, 59.69) -> (74.51, 59.6138) centre (74.5862, 59.6138) ccw
  line L862 (79.336, 73.9902) -> (79.336, 74.8538)
  arc A533 (73.7498, 58.674) -> (73.826, 58.7502) centre (73.7498, 58.7502) ccw
  line L863 (72.1732, 78.613) -> (73.0368, 78.613)
  arc A534 (69.0762, 68.16) -> (69, 68.0838) centre (69.0762, 68.0838) ccw
  line L864 (73.826, 58.7502) -> (73.826, 59.6138)
  arc A535 (59.828, 57.642) -> (59.723, 57.747) centre (59.723, 57.642) ccw
  line L865 (58.028, 60.642) -> (58.028, 59.452)
  arc A536 (77.04, 58.7502) -> (77.1162, 58.674) centre (77.1162, 58.7502) ccw
  line L866 (69.0762, 65.444) -> (69.9398, 65.444)
  line L867 (78.74, 59.6138) -> (78.74, 58.7502)
  line L868 (73.0368, 79.629) -> (72.1732, 79.629)
  arc A537 (73.826, 59.6138) -> (73.7498, 59.69) centre (73.7498, 59.6138) ccw
  line L869 (48.475, 76.0222) -> (48.475, 76.8858)
  arc A538 (75.4498, 58.674) -> (75.526, 58.7502) centre (75.4498, 58.7502) ccw
  line L870 (79.6798, 59.69) -> (78.8162, 59.69)
  line L871 (74.5862, 58.674) -> (75.4498, 58.674)
  arc A539 (58.133, 60.747) -> (58.028, 60.642) centre (58.133, 60.642) ccw
  arc A540 (69.0762, 66.46) -> (69, 66.3838) centre (69.0762, 66.3838) ccw
  arc A541 (79.6798, 58.674) -> (79.756, 58.7502) centre (79.6798, 58.7502) ccw
  line L872 (77.9798, 59.69) -> (77.1162, 59.69)
  line L873 (69.0762, 67.144) -> (69.9398, 67.144)
  arc A542 (79.756, 59.6138) -> (79.6798, 59.69) centre (79.6798, 59.6138) ccw
  arc A543 (72.097, 78.6892) -> (72.1732, 78.613) centre (72.1732, 78.6892) ccw
  line L874 (47.459, 76.8858) -> (47.459, 76.0222)
  arc A544 (76.6962, 74.93) -> (76.62, 74.8538) centre (76.6962, 74.8538) ccw
  arc A545 (71.3368, 78.613) -> (71.413, 78.6892) centre (71.3368, 78.6892) ccw
  line L875 (70.4732, 78.613) -> (71.3368, 78.613)
  arc A546 (70.4732, 79.629) -> (70.397, 79.5528) centre (70.4732, 79.5528) ccw
  line L876 (48.3988, 76.962) -> (47.5352, 76.962)
  arc A547 (62.23, 72.1088) -> (62.1538, 72.185) centre (62.1538, 72.1088) ccw
  arc A548 (73.113, 79.5528) -> (73.0368, 79.629) centre (73.0368, 79.5528) ccw
  line L877 (75.526, 58.7502) -> (75.526, 59.6138)
  line L878 (58.133, 56.347) -> (59.723, 56.347)
  line L879 (46.775, 76.0222) -> (46.775, 76.8858)
  arc A549 (72.81, 58.7502) -> (72.8862, 58.674) centre (72.8862, 58.7502) ccw
  line L880 (77.5598, 74.93) -> (76.6962, 74.93)
  line L881 (73.7498, 59.69) -> (72.8862, 59.69)
  line L882 (58.028, 57.642) -> (58.028, 56.452)
  arc A550 (70.016, 66.3838) -> (69.9398, 66.46) centre (69.9398, 66.3838) ccw
  line L883 (61.2902, 69.469) -> (62.1538, 69.469)
  arc A551 (59.723, 59.347) -> (59.828, 59.452) centre (59.723, 59.452) ccw
  line L884 (70.397, 79.5528) -> (70.397, 78.6892)
  line L885 (69.9398, 68.16) -> (69.0762, 68.16)
  line L886 (74.51, 59.6138) -> (74.51, 58.7502)
  arc A552 (72.8862, 59.69) -> (72.81, 59.6138) centre (72.8862, 59.6138) ccw
  line L887 (111.905, 56.1) -> (113.095, 56.1)
  arc A553 (116.2, 57.795) -> (116.095, 57.9) centre (116.095, 57.795) ccw
  arc A554 (116.095, 56.1) -> (116.2, 56.205) centre (116.095, 56.205) ccw
  arc A555 (54.7, 55.295) -> (54.595, 55.4) centre (54.595, 55.295) ccw
  line L888 (82.0928, 61.888) -> (81.2292, 61.888)
  line L889 (113.095, 57.9) -> (111.905, 57.9)
  arc A556 (81.153, 70.2192) -> (81.2292, 70.143) centre (81.2292, 70.2192) ccw
  line L890 (114.905, 56.1) -> (116.095, 56.1)
  line L891 (81.2292, 62.572) -> (82.0928, 62.572)
  arc A557 (74.51, 58.7502) -> (74.5862, 58.674) centre (74.5862, 58.7502) ccw
  arc A558 (81.153, 62.6482) -> (81.2292, 62.572) centre (81.2292, 62.6482) ccw
  arc A559 (58.133, 57.747) -> (58.028, 57.642) centre (58.133, 57.642) ccw
  arc A560 (69, 67.2202) -> (69.0762, 67.144) centre (69.0762, 67.2202) ccw
  arc A561 (51.7, 55.295) -> (51.595, 55.4) centre (51.595, 55.295) ccw
  line L892 (59.828, 59.452) -> (59.828, 60.642)
  line L893 (70.016, 65.5202) -> (70.016, 66.3838)
  arc A562 (111.8, 56.205) -> (111.905, 56.1) centre (111.905, 56.205) ccw
  line L894 (75.4498, 59.69) -> (74.5862, 59.69)
  arc A563 (82.0928, 71.843) -> (82.169, 71.9192) centre (82.0928, 71.9192) ccw
  line L895 (59.723, 60.747) -> (58.133, 60.747)
  arc A564 (79.2598, 73.914) -> (79.336, 73.9902) centre (79.2598, 73.9902) ccw
  line L896 (59.723, 57.747) -> (58.133, 57.747)
  arc A565 (75.526, 59.6138) -> (75.4498, 59.69) centre (75.4498, 59.6138) ccw
  line L897 (111.8, 57.795) -> (111.8, 56.205)
  arc A566 (82.169, 72.7828) -> (82.0928, 72.859) centre (82.0928, 72.7828) ccw
  line L898 (81.153, 72.7828) -> (81.153, 71.9192)
  arc A567 (81.2292, 71.159) -> (81.153, 71.0828) centre (81.2292, 71.0828) ccw
  arc A568 (50.3, 53.705) -> (50.405, 53.6) centre (50.405, 53.705) ccw
  line L899 (50.405, 53.6) -> (51.595, 53.6)
  line L900 (81.2292, 60.872) -> (82.0928, 60.872)
  arc A569 (114.8, 56.205) -> (114.905, 56.1) centre (114.905, 56.205) ccw
  arc A570 (59.723, 56.347) -> (59.828, 56.452) centre (59.723, 56.452) ccw
  arc A571 (81.153, 60.9482) -> (81.2292, 60.872) centre (81.2292, 60.9482) ccw
  arc A572 (111.905, 57.9) -> (111.8, 57.795) centre (111.905, 57.795) ccw
  line L901 (51.595, 55.4) -> (50.405, 55.4)
  arc A573 (82.169, 71.0828) -> (82.0928, 71.159) centre (82.0928, 71.0828) ccw
  arc A574 (82.0928, 60.872) -> (82.169, 60.9482) centre (82.0928, 60.9482) ccw
  line L902 (82.169, 71.9192) -> (82.169, 72.7828)
  arc A575 (78.3962, 74.93) -> (78.32, 74.8538) centre (78.3962, 74.8538) ccw
  line L903 (81.2292, 71.843) -> (82.0928, 71.843)
  line L904 (82.0928, 72.859) -> (81.2292, 72.859)
  line L905 (81.2292, 70.143) -> (82.0928, 70.143)
  arc A576 (76.62, 73.9902) -> (76.6962, 73.914) centre (76.6962, 73.9902) ccw
  line L906 (82.0928, 63.588) -> (81.2292, 63.588)
  line L907 (59.828, 56.452) -> (59.828, 57.642)
  arc A577 (77.9798, 58.674) -> (78.056, 58.7502) centre (77.9798, 58.7502) ccw
  arc A578 (114.905, 57.9) -> (114.8, 57.795) centre (114.905, 57.795) ccw
  line L908 (53.3, 55.295) -> (53.3, 53.705)
  arc A579 (53.3, 53.705) -> (53.405, 53.6) centre (53.405, 53.705) ccw
  arc A580 (58.028, 56.452) -> (58.133, 56.347) centre (58.133, 56.452) ccw
  line L909 (72.81, 59.6138) -> (72.81, 58.7502)
  line L910 (116.2, 56.205) -> (116.2, 57.795)
  line L911 (69.9398, 66.46) -> (69.0762, 66.46)
  line L912 (78.32, 74.8538) -> (78.32, 73.9902)
  line L913 (81.153, 71.0828) -> (81.153, 70.2192)
  arc A581 (53.405, 55.4) -> (53.3, 55.295) centre (53.405, 55.295) ccw
  line L914 (58.133, 59.347) -> (59.723, 59.347)
  arc A582 (69, 65.5202) -> (69.0762, 65.444) centre (69.0762, 65.5202) ccw
  arc A583 (51.595, 53.6) -> (51.7, 53.705) centre (51.595, 53.705) ccw
  arc A584 (82.0928, 70.143) -> (82.169, 70.2192) centre (82.0928, 70.2192) ccw
  line L915 (69, 68.0838) -> (69, 67.2202)
  line L916 (76.6962, 73.914) -> (77.5598, 73.914)
  line L917 (69, 66.3838) -> (69, 65.5202)
  line L918 (82.169, 62.6482) -> (82.169, 63.5118)
  line L919 (50.5682, 82.842) -> (51.4318, 82.842)
  arc A585 (81.2292, 63.588) -> (81.153, 63.5118) centre (81.2292, 63.5118) ccw
  arc A586 (51.4318, 82.842) -> (51.508, 82.9182) centre (51.4318, 82.9182) ccw
  line L920 (116.095, 57.9) -> (114.905, 57.9)
  line L921 (51.7, 53.705) -> (51.7, 55.295)
  line L922 (43.815, 85.6878) -> (43.815, 84.8242)
  arc A587 (82.0928, 62.572) -> (82.169, 62.6482) centre (82.0928, 62.6482) ccw
  line L923 (82.169, 60.9482) -> (82.169, 61.8118)
  arc A588 (51.4318, 81.142) -> (51.508, 81.2182) centre (51.4318, 81.2182) ccw
  arc A589 (44.831, 87.3878) -> (44.7548, 87.464) centre (44.7548, 87.3878) ccw
  arc A590 (54.008, 87.7818) -> (53.9318, 87.858) centre (53.9318, 87.7818) ccw
  line L924 (51.508, 81.2182) -> (51.508, 82.0818)
  line L925 (82.0928, 71.159) -> (81.2292, 71.159)
  arc A591 (54.595, 53.6) -> (54.7, 53.705) centre (54.595, 53.705) ccw
  arc A592 (51.508, 82.0818) -> (51.4318, 82.158) centre (51.4318, 82.0818) ccw
  arc A593 (51.508, 83.7818) -> (51.4318, 83.858) centre (51.4318, 83.7818) ccw
  line L926 (43.815, 87.3878) -> (43.815, 86.5242)
  arc A594 (50.405, 55.4) -> (50.3, 55.295) centre (50.405, 55.295) ccw
  line L927 (44.831, 86.5242) -> (44.831, 87.3878)
  line L928 (54.7, 53.705) -> (54.7, 55.295)
  line L929 (113.2, 56.205) -> (113.2, 57.795)
  arc A595 (81.2292, 61.888) -> (81.153, 61.8118) centre (81.2292, 61.8118) ccw
  line L930 (74.5862, 73.914) -> (75.4498, 73.914)
  line L931 (81.153, 61.8118) -> (81.153, 60.9482)
  arc A596 (43.815, 86.5242) -> (43.8912, 86.448) centre (43.8912, 86.5242) ccw
  line L932 (53.405, 53.6) -> (54.595, 53.6)
  line L933 (52.992, 86.0818) -> (52.992, 85.2182)
  arc A597 (43.815, 84.8242) -> (43.8912, 84.748) centre (43.8912, 84.8242) ccw
  line L934 (82.169, 70.2192) -> (82.169, 71.0828)
  arc A598 (50.492, 82.9182) -> (50.5682, 82.842) centre (50.5682, 82.9182) ccw
  line L935 (114.8, 57.795) -> (114.8, 56.205)
  line L936 (75.526, 73.9902) -> (75.526, 74.8538)
  line L937 (54.008, 86.9182) -> (54.008, 87.7818)
  arc A599 (54.008, 86.0818) -> (53.9318, 86.158) centre (53.9318, 86.0818) ccw
  line L938 (50.492, 82.0818) -> (50.492, 81.2182)
  arc A600 (53.9318, 86.842) -> (54.008, 86.9182) centre (53.9318, 86.9182) ccw
  line L939 (44.7548, 85.764) -> (43.8912, 85.764)
  arc A601 (53.0682, 86.158) -> (52.992, 86.0818) centre (53.0682, 86.0818) ccw
  line L940 (51.4318, 83.858) -> (50.5682, 83.858)
  arc A602 (82.169, 63.5118) -> (82.0928, 63.588) centre (82.0928, 63.5118) ccw
  line L941 (50.5682, 81.142) -> (51.4318, 81.142)
  line L942 (50.492, 83.7818) -> (50.492, 82.9182)
  line L943 (44.831, 84.8242) -> (44.831, 85.6878)
  line L944 (51.508, 82.9182) -> (51.508, 83.7818)
  line L945 (54.595, 55.4) -> (53.405, 55.4)
  arc A603 (73.826, 74.8538) -> (73.7498, 74.93) centre (73.7498, 74.8538) ccw
  arc A604 (113.2, 57.795) -> (113.095, 57.9) centre (113.095, 57.795) ccw
  arc A605 (53.9318, 85.142) -> (54.008, 85.2182) centre (53.9318, 85.2182) ccw
  arc A606 (77.5598, 73.914) -> (77.636, 73.9902) centre (77.5598, 73.9902) ccw
  line L946 (73.7498, 74.93) -> (72.8862, 74.93)
  arc A607 (44.831, 85.6878) -> (44.7548, 85.764) centre (44.7548, 85.6878) ccw
  arc A608 (82.169, 61.8118) -> (82.0928, 61.888) centre (82.0928, 61.8118) ccw
  line L947 (81.153, 63.5118) -> (81.153, 62.6482)
  arc A609 (72.8862, 74.93) -> (72.81, 74.8538) centre (72.8862, 74.8538) ccw
  line L948 (50.3, 55.295) -> (50.3, 53.705)
  arc A610 (81.153, 71.9192) -> (81.2292, 71.843) centre (81.2292, 71.9192) ccw
  arc A611 (50.5682, 82.158) -> (50.492, 82.0818) centre (50.5682, 82.0818) ccw
  line L949 (74.51, 74.8538) -> (74.51, 73.9902)
  arc A612 (75.4498, 73.914) -> (75.526, 73.9902) centre (75.4498, 73.9902) ccw
  arc A613 (73.7498, 73.914) -> (73.826, 73.9902) centre (73.7498, 73.9902) ccw
  line L950 (53.0682, 86.842) -> (53.9318, 86.842)
  arc A614 (74.51, 73.9902) -> (74.5862, 73.914) centre (74.5862, 73.9902) ccw
  line L951 (72.8862, 73.914) -> (73.7498, 73.914)
  arc A615 (113.095, 56.1) -> (113.2, 56.205) centre (113.095, 56.205) ccw
  arc A616 (124.8453, 94.5778) -> (124.7691, 94.654) centre (124.7691, 94.5778) ccw
  arc A617 (90.717, 91.6178) -> (90.6408, 91.694) centre (90.6408, 91.6178) ccw
  arc A618 (74.5862, 74.93) -> (74.51, 74.8538) centre (74.5862, 74.8538) ccw
  line L952 (53.9318, 87.858) -> (53.0682, 87.858)
  line L953 (92.417, 90.7542) -> (92.417, 91.6178)
  arc A619 (90.6408, 90.678) -> (90.717, 90.7542) centre (90.6408, 90.7542) ccw
  arc A620 (110.3673, 94.2458) -> (110.2911, 94.322) centre (110.2911, 94.2458) ccw
  line L954 (110.2911, 94.322) -> (109.4275, 94.322)
  line L955 (123.8293, 94.5778) -> (123.8293, 93.7142)
  line L956 (54.008, 85.2182) -> (54.008, 86.0818)
  line L957 (90.6408, 91.694) -> (89.7772, 91.694)
  line L958 (110.2911, 92.622) -> (109.4275, 92.622)